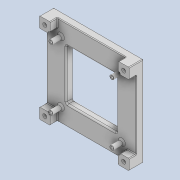
# Autodesk Inventor part: Back_Plate
Saved by Autodesk Inventor 2020 (Build 240168000, 168)
## iProperties
Created: 2020-08-27
Part Number: Back_Plate
Material: Generic
Document SubType Name: Modeling
Designer: conno
Density: 1 g/cm^3
Appearance: Default
Author: conno
Autodesk Inventor part; units mm, degrees
ref_plane "YZ Plane" through (0, 0, 0) normal (1, 0, 0) x (0, 1, 0)
ref_plane "XZ Plane" through (0, 0, 0) normal (0, 1, 0) x (-1, 0, 0)
ref_plane "XY Plane" through (0, 0, 0) normal (0, 0, 1) x (1, 0, 0)
sketch "Sketch1" plane through (0, 0, 0) normal (0, 0, 1) x (1, 0, 0)
  line L0 (-62.5, -62.5) -> (62.5, -62.5)
  line L1 (62.5, -62.5) -> (62.5, 62.5)
  line L2 (62.5, 62.5) -> (-62.5, 62.5)
  line L3 (-62.5, 62.5) -> (-62.5, -62.5)
  line L4 (-62.5, -62.5) -> (62.5, 62.5) construction
  line L5 (62.5, -62.5) -> (-62.5, 62.5) construction
  point P0 (0, 0)
  dimension "d0" = 125
  dimension "d1" = 125
  constraints: 12 end point, 2 midpoint, 2 parallel, 1 horizontal, 1 perpendicular
  measures "d0" distance of L2.end L1.end
  measures "d1" distance of L2.end L0.start
extrude "Extrusion1" add sketch "Sketch1" along normal blind 10
sketch "Sketch2" plane through (0, 0, 10) normal (0, 0, 1) x (1, 0, 0)
  circle A0 centre (-42.5, 42.5) radius 2.875
  circle A1 centre (-42.5, 42.5) radius 1.4
  circle A2 centre (42.5, 42.5) radius 2.875
  circle A3 centre (42.5, 42.5) radius 1.4
  circle A4 centre (-42.5, -42.5) radius 2.875
  circle A5 centre (42.5, -42.5) radius 2.875
  circle A6 centre (-42.5, -42.5) radius 1.4
  circle A7 centre (42.5, -42.5) radius 1.4
  point P0 (0, 0)
  dimension "d4" = 5.75
  dimension "d5" = 42.5
  dimension "d6" = 42.5
  dimension "d7" = 2.8
  dimension "d8" = 5.75
  dimension "d9" = 85
  dimension "d10" = 2.8
  dimension "d11" = 42.5
  dimension "d12" = 5.75
  dimension "d13" = 5.75
  dimension "d14" = 85
  dimension "d15" = 0
  dimension "d16" = 85
  dimension "d17" = 0
  dimension "d18" = 2.8
  dimension "d19" = 2.8
  constraints: 8 centre point, 4 coincident
  measures "d4" diameter of A0
  measures "d5" horizontal distance of point (0, 0) A0.centre
  measures "d6" horizontal distance of point (0, 0) A0.centre
  measures "d7" diameter of A1
  measures "d8" diameter of A2
  measures "d9" distance of A2.centre A0.centre
  measures "d10" diameter of A3
  measures "d11" horizontal distance of point (0, 0) A2.centre
  measures "d12" diameter of A4
  measures "d13" diameter of A5
  measures "d14" distance of A4.centre A0.centre
  measures "d15" horizontal distance of A0.centre A4.centre
  measures "d16" distance of A4.centre A5.centre
  measures "d17" vertical distance of A4.centre A5.centre
  measures "d18" diameter of A6
  measures "d19" diameter of A7
extrude "Extrusion2" add sketch "Sketch2" along normal blind 14
sketch "Sketch3" plane through (0, 0, 10) normal (0, 0, 1) x (1, 0, 0)
  line L0 (-35, -35) -> (35, -35)
  line L1 (35, -35) -> (35, 35)
  line L2 (35, 35) -> (-35, 35)
  line L3 (-35, 35) -> (-35, -35)
  line L4 (-35, -35) -> (35, 35) construction
  line L5 (35, -35) -> (-35, 35) construction
  point P0 (0, 0)
  dimension "d22" = 70
  dimension "d23" = 70
  constraints: 12 end point, 2 midpoint, 2 parallel, 1 horizontal, 1 perpendicular
  measures "d22" distance of L2.end L1.end
  measures "d23" distance of L1.end L0.end
extrude "Extrusion3" cut sketch "Sketch3" against normal through all
sketch "Sketch4" plane through (0, 0, 10) normal (0, 0, 1) x (1, 0, 0)
  line L0 (62.5, 62.5) -> (-62.5, 62.5) projected
  line L1 (-62.5, 62.5) -> (-47.5, 62.5)
  line L2 (-47.5, 62.5) -> (-47.5, 47.5)
  line L3 (-47.5, 47.5) -> (-62.5, 47.5)
  line L4 (-62.5, 47.5) -> (-62.5, 62.5)
  line L5 (62.5, 62.5) -> (47.5, 62.5)
  line L6 (47.5, 62.5) -> (47.5, 47.5)
  line L7 (47.5, 47.5) -> (62.5, 47.5)
  line L8 (62.5, 47.5) -> (62.5, 62.5)
  line L9 (62.5, -62.5) -> (62.5, 62.5) projected
  line L10 (62.5, -62.5) -> (47.5, -62.5)
  line L11 (47.5, -62.5) -> (47.5, -47.5)
  line L12 (47.5, -47.5) -> (62.5, -47.5)
  line L13 (62.5, -47.5) -> (62.5, -62.5)
  line L14 (-62.5, 62.5) -> (-62.5, -62.5) projected
  line L15 (-62.5, -62.5) -> (-47.5, -62.5)
  line L16 (-47.5, -62.5) -> (-47.5, -47.5)
  line L17 (-47.5, -47.5) -> (-62.5, -47.5)
  line L18 (-62.5, -47.5) -> (-62.5, -62.5)
  point P0 (0, 0)
  point P1 (-62.5, -47.5)
  dimension "d27" = 15
  dimension "d28" = 15
  dimension "d29" = 15
  dimension "d30" = 15
  dimension "d31" = 15
  dimension "d32" = 15
  dimension "d33" = 15
  dimension "d34" = 15
  constraints: 32 end point, 8 parallel, 4 horizontal, 4 perpendicular
  measures "d27" distance of L2.end L3.end
  measures "d28" distance of L1.end L2.end
  measures "d29" distance of L7.end L6.end
  measures "d30" distance of L6.end L5.end
  measures "d31" distance of L11.end L12.end
  measures "d32" distance of L10.end L11.end
  measures "d33" distance of L17.end L16.end
  measures "d34" distance of L16.end L15.end
extrude "Extrusion4" add sketch "Sketch4" along normal blind 10
sketch "Sketch5" plane through (0, 0, 0) normal (0, 0, -1) x (-1, 0, 0)
  circle A0 centre (-55, 55) radius 5
  line L0 (-62.5, 62.5) -> (62.5, 62.5) projected
  line L1 (-62.5, -62.5) -> (-62.5, 62.5) projected
  circle A1 centre (55, 55) radius 5
  line L2 (62.5, 62.5) -> (62.5, -62.5) projected
  circle A2 centre (-55, -55) radius 5
  circle A3 centre (55, -55) radius 5
  line L3 (62.5, -62.5) -> (-62.5, -62.5) projected
  point P0 (0, 0)
  dimension "d37" = 10
  dimension "d38" = 7.5
  dimension "d39" = 7.5
  dimension "d40" = 10
  dimension "d41" = 7.5
  dimension "d42" = 7.5
  dimension "d43" = 10
  dimension "d44" = 10
  dimension "d45" = 7.5
  dimension "d46" = 7.5
  dimension "d47" = 7.5
  dimension "d48" = 7.5
  constraints: 4 centre point
  measures "d37" diameter of A0
  measures "d38" distance from line of L0 A0.centre
  measures "d39" distance from line of L1 A0.centre
  measures "d40" diameter of A1
  measures "d41" distance from line of L0 A1.centre
  measures "d42" distance from line of L2 A1.centre
  measures "d43" diameter of A2
  measures "d44" diameter of A3
  measures "d45" distance from line of L3 A2.centre
  measures "d46" distance from line of L1 A2.centre
  measures "d47" distance from line of L2 A3.centre
  measures "d48" distance from line of L3 A3.centre
extrude "Extrusion5" cut sketch "Sketch5" against normal blind 15 contours A0 | A1 | A2 | A3
sketch "Sketch6" plane through (55, 55, 15) normal (0, 0, -1) x (-1, 0, 0)
  point P0 (55, -55)
  point P1 (0, 0)
hole "Hole1" at (55, 55, 15) direction (0, 0, 1) diameter 5.5 end through all clearance for "Flat Head Machine Screw" size "M5" standard "Ansi Metric M Profile"
sketch "Sketch7" plane through (-55, 55, 15) normal (0, 0, -1) x (-1, 0, 0)
  point P0 (-55, -55)
  point P1 (0, 0)
hole "Hole2" at (-55, 55, 15) direction (0, 0, 1) diameter 5.5 end through all clearance for "Flat Head Machine Screw" size "M5" standard "Ansi Metric M Profile"
sketch "Sketch8" plane through (55, -55, 15) normal (0, 0, -1) x (-1, 0, 0)
  point P0 (55, 55)
  point P1 (0, 0)
hole "Hole3" at (55, -55, 15) direction (0, 0, 1) diameter 5.5 end through all clearance for "Flat Head Machine Screw" size "M5" standard "Ansi Metric M Profile"
sketch "Sketch9" plane through (-55, -55, 15) normal (0, 0, -1) x (-1, 0, 0)
  point P0 (-55, 55)
  point P1 (0, 0)
hole "Hole4" at (-55, -55, 15) direction (0, 0, 1) diameter 5.5 end through all clearance for "Flat Head Machine Screw" size "M5" standard "Ansi Metric M Profile"
fillet "Fillet2" radius 2 12 edges at (-35, -35, 5) (-35, 0, 10) (-35, 0, 0) (0, -35, 10) (0, -35, 0) (35, -35, 5) (35, 0, 0) (35, 0, 10) (35, 35, 5) (0, 35, 0) (0, 35, 10) (-35, 35, 5)
chamfer "Chamfer1" distance 0.5 angle 45 4 edges at (-43.9, -42.5, 24) (-43.9, 42.5, 24) (41.1, -42.5, 24) (41.1, 42.5, 24)
chamfer "Chamfer2" distance 1.5 angle 45 4 edges at (55, -57.75, 15) (-55, -57.75, 15) (55, 52.25, 15) (-55, 52.25, 15)
fillet "Fillet5" radius 2 4 edges at (39.625, -42.5, 10) (39.625, 42.5, 10) (-45.375, -42.5, 10) (-45.375, 42.5, 10)
sketch "Sketch12" plane through (-62.5, -62.5, 0) normal (0, -1, 0) x (1, 0, 0)
  circle A0 centre (62.5, 5) radius 2.54
  line L0 (0, 0) -> (0, 20) projected
  point P0 (62.5, 0)
  dimension "d91" = 5.08
  dimension "d92" = 5
  dimension "d93" = 62.5
  constraints: 1 centre point
  measures "d91" diameter of A0
  measures "d92" distance of point (62.5, 0) A0.centre
  measures "d93" distance from line of L0 A0.centre
extrude "Extrusion6" cut sketch "Sketch12" against normal blind 12.7
sketch "Sketch16" plane through (0, 0, 20) normal (0, 0, 1) x (1, 0, 0)
  line L0 (49, -50) -> (47.5, -50)
  arc A0 (49, -50) -> (50, -49) centre (49, -49) ccw
  line L1 (50, -47.5) -> (50, -49)
  line L2 (50, -47.5) -> (47.5, -47.5)
  line L3 (47.5, -47.5) -> (47.5, -50)
  line L4 (47.5, -47.5) -> (47.5, -62.5) projected
  line L5 (47.5, 50) -> (49, 50)
  line L6 (47.5, 50) -> (47.5, 47.5)
  arc A1 (50, 49) -> (49, 50) centre (49, 49) ccw
  line L7 (50, 49) -> (50, 47.5)
  line L8 (47.5, 47.5) -> (50, 47.5)
  line L9 (47.5, 62.5) -> (47.5, 47.5) projected
  line L10 (-47.5, 47.5) -> (-47.5, 62.5) projected
  line L11 (-62.5, -47.5) -> (-47.5, -47.5) projected
  arc A2 (-49, 50) -> (-50, 49) centre (-49, 49) ccw
  line L12 (-49, 50) -> (-47.5, 50)
  line L13 (-47.5, 47.5) -> (-47.5, 50)
  line L14 (-50, 47.5) -> (-47.5, 47.5)
  line L15 (-50, 47.5) -> (-50, 49)
  arc A3 (-50, -49) -> (-49, -50) centre (-49, -49) ccw
  line L16 (-47.5, -50) -> (-49, -50)
  line L17 (-47.5, -50) -> (-47.5, -47.5)
  line L18 (-47.5, -47.5) -> (-50, -47.5)
  line L19 (-50, -49) -> (-50, -47.5)
  point P0 (0, 0)
  constraints: 32 end point, 8 point on circle, 4 centre point
extrude "Extrusion7" cut sketch "Sketch16" against normal up to surface (10 mm away)
fillet "Fillet7" radius 1 8 edges at (-50, -47.5, 15) (-47.5, -50, 15) (-50, 47.5, 15) (-47.5, 50, 15) (47.5, 50, 15) (50, 47.5, 15) (50, -47.5, 15) (47.5, -50, 15)
fillet "Fillet8" radius 1 48 edges at (47.7929, 50.2929, 10) (48.75, 50, 10) (49.7071, 49.7071, 10) (50, 48.75, 10) (50.2929, 47.7929, 10) (56.75, 47.5, 10) (47.5, 56.75, 10) (0, 62.5, 10) (47.5, 62.5, 15) (62.5, 47.5, 15) (62.5, 0, 10) (62.5, 62.5, 10) (62.5, 0, 0) (0, 62.5, 0) (50.2929, -47.7929, 10) (50, -48.75, 10) (49.7071, -49.7071, 10) (48.75, -50, 10) (47.7929, -50.2929, 10) (47.5, -56.75, 10) (56.75, -47.5, 10) (62.5, -47.5, 15) (62.5, -62.5, 10) (-47.7929, 50.2929, 10) (-48.75, 50, 10) (-49.7071, 49.7071, 10) (-50, 48.75, 10) (-50.2929, 47.7929, 10) (-56.75, 47.5, 10) (-47.5, 56.75, 10) (-47.5, 62.5, 15) (-62.5, 62.5, 10) (-62.5, 47.5, 15) (-62.5, 0, 10) (-62.5, 0, 0) (-62.5, -47.5, 15) (-62.5, -62.5, 10) (-47.5, -62.5, 15) (0, -62.5, 10) (47.5, -62.5, 15) (-47.7929, -50.2929, 10) (-48.75, -50, 10) (-49.7071, -49.7071, 10) (-50, -48.75, 10) (-50.2929, -47.7929, 10) (-56.75, -47.5, 10) (-47.5, -56.75, 10) (0, -62.5, 0)
equation "\"d105\" = 55deg"
equation "\"Sketch13_Pitch\" = 1.27"
body "Solid1"
